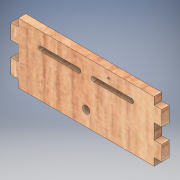
# Autodesk Inventor part: EndPulleyMount
Saved by Autodesk Inventor 2019 (Build 230136000, 136)
## iProperties
Created: 2019-01-17
Part Number: EndPulleyMount
Material: Wood (Birch)
Document SubType Name: Modeling
Designer: nxgam
Density: 0.55 g/cm^3
Appearance: Birch - Natural Polished
Author: nxgam
Autodesk Inventor part; units mm, degrees
ref_plane "YZ Plane" through (0, 0, 0) normal (1, 0, 0) x (0, 1, 0)
ref_plane "XZ Plane" through (0, 0, 0) normal (0, 1, 0) x (-1, 0, 0)
ref_plane "XY Plane" through (0, 0, 0) normal (0, 0, 1) x (1, 0, 0)
sketch "Sketch1" plane through (0, 0, 0) normal (0, 0, 1) x (1, 0, 0)
  line L0 (45.72, 0) -> (45.72, 40.64)
  line L1 (45.72, 40.64) -> (-45.72, 40.64)
  line L2 (-45.72, 40.64) -> (-45.72, 9.301)
  line L3 (-45.72, 5.08) -> (-50.8, 5.08)
  line L4 (-50.8, 5.08) -> (-50.8, 15.24)
  line L5 (-50.8, 15.24) -> (-45.72, 15.24)
  line L6 (-45.72, 15.24) -> (-45.72, 5.08)
  line L7 (-45.72, 25.4) -> (-50.8, 25.4)
  line L8 (-50.8, 25.4) -> (-50.8, 35.56)
  line L9 (-50.8, 35.56) -> (-45.72, 35.56)
  line L10 (-45.72, 35.56) -> (-45.72, 25.4)
  line L11 (-45.72, 45.72) -> (-50.8, 45.72)
  line L12 (-50.8, 45.72) -> (-50.8, 55.88)
  line L13 (-50.8, 55.88) -> (-45.72, 55.88)
  line L14 (-45.72, 55.88) -> (-45.72, 45.72)
  line L15 (0, 40.64) -> (0, 0) construction
  line L16 (45.72, 40.64) -> (45.72, 0)
  line L17 (45.72, 5.08) -> (50.8, 5.08)
  line L18 (50.8, 5.08) -> (50.8, 15.24)
  line L19 (50.8, 15.24) -> (45.72, 15.24)
  line L20 (45.72, 15.24) -> (45.72, 5.08)
  line L21 (45.72, 25.4) -> (50.8, 25.4)
  line L22 (50.8, 25.4) -> (50.8, 35.56)
  line L23 (50.8, 35.56) -> (45.72, 35.56)
  line L24 (45.72, 35.56) -> (45.72, 25.4)
  line L25 (45.72, 45.72) -> (50.8, 45.72)
  line L26 (50.8, 45.72) -> (50.8, 55.88)
  line L27 (50.8, 55.88) -> (45.72, 55.88)
  line L28 (45.72, 55.88) -> (45.72, 45.72)
  line L29 (-45.72, 5.08) -> (-45.72, 0)
  line L30 (-45.72, 0) -> (45.72, 0)
  line L31 (45.72, 40.64) -> (-45.72, 40.64)
  line L32 (-45.72, 40.64) -> (-45.72, 0)
  line L33 (-45.72, 0) -> (45.72, 0)
  line L34 (45.72, 0) -> (45.72, 40.64)
  dimension "d0" = 91.44
  dimension "d2" = 10.16
  dimension "d3" = 5.08
  dimension "d7" = 20.32
  dimension "d14" = 5.08
  dimension "d15" = 40.64
  constraints: 70 end point, 12 symmetric about line, 5 parallel, 4 perpendicular, 3 vertical, 2 horizontal, 2 midpoint, 2 point on line, 1 coincident, 16 other
  measures "d0" distance of L1.end L0.end
  measures "d2" distance of L3.end L4.end
  measures "d3" distance of L4.end L5.end
  measures "d7" distance of L3.start L7.start
  measures "d14" distance of L3.start L29.end
  measures "d15" distance between parallel lines of L30 L1
extrude "Extrusion2" add sketch "Sketch1" along normal blind 5.08 contours L30 L29 L6 L2 L1 L0 | L0 L19 L18 L17 | L3 L4 L5 L2 L6 | L0 L23 L22 L21 | L7 L8 L9 L2
sketch "Sketch4" plane through (0, 0, 5.08) normal (0, 0, 1) x (1, 0, 0)
  line L0 (45.72, 40.64) -> (-45.72, 40.64) construction
  line L1 (-30.48, 30.48) -> (-5.08, 30.48)
  line L2 (-30.48, 28.98) -> (-5.08, 28.98)
  line L3 (-5.08, 31.98) -> (-30.48, 31.98)
  arc A0 (-30.48, 31.98) -> (-30.48, 28.98) centre (-30.48, 30.48) ccw
  arc A1 (-5.08, 28.98) -> (-5.08, 31.98) centre (-5.08, 30.48) ccw
  line L4 (30.48, 30.48) -> (5.08, 30.48)
  line L5 (30.48, 28.98) -> (5.08, 28.98)
  line L6 (5.08, 31.98) -> (30.48, 31.98)
  arc A2 (30.48, 28.98) -> (30.48, 31.98) centre (30.48, 30.48) ccw
  arc A3 (5.08, 31.98) -> (5.08, 28.98) centre (5.08, 30.48) ccw
  line L7 (-50.8, 25.4) -> (-45.72, 25.4) projected
  line L8 (-45.72, 25.4) -> (-45.72, 15.24) projected
  line L9 (-45.72, 15.24) -> (-50.8, 15.24) projected
  line L10 (-50.8, 15.24) -> (-50.8, 5.08) projected
  line L11 (-50.8, 5.08) -> (-45.72, 5.08) projected
  line L12 (-45.72, 5.08) -> (-45.72, 0) projected
  line L13 (-45.72, 0) -> (45.72, 0) projected
  line L14 (45.72, 0) -> (45.72, 5.08) projected
  line L15 (45.72, 5.08) -> (50.8, 5.08) projected
  line L16 (50.8, 5.08) -> (50.8, 15.24) projected
  line L17 (50.8, 15.24) -> (45.72, 15.24) projected
  line L18 (45.72, 15.24) -> (45.72, 25.4) projected
  line L19 (45.72, 25.4) -> (50.8, 25.4) projected
  line L20 (50.8, 25.4) -> (50.8, 35.56) projected
  line L21 (50.8, 35.56) -> (45.72, 35.56) projected
  line L22 (45.72, 35.56) -> (45.72, 40.64) projected
  line L23 (45.72, 40.64) -> (-45.72, 40.64) projected
  line L24 (-45.72, 40.64) -> (-45.72, 35.56) projected
  line L25 (-45.72, 35.56) -> (-50.8, 35.56) projected
  line L26 (-50.8, 35.56) -> (-50.8, 25.4) projected
  line L27 (0, 40.64) -> (0, 0) construction
  circle A4 centre (0, 10.16) radius 2.5
  point P0 (-17.78, 30.48)
  point P1 (17.78, 30.48)
  point P2 (17.78, 30.48)
  dimension "d25" = 3
  dimension "d26" = 25.4
  dimension "d32" = 17.78
  dimension "d33" = 17.78
  dimension "d34" = 25.4
  dimension "d35" = 10.16
  dimension "d36" = 1.5
  dimension "d37" = 1.5
  dimension "d38" = 5
  dimension "d39" = 10.16
  constraints: 18 end point, 8 point on circle, 8 tangent, 5 centre point, 3 midpoint, 1 coincident, 1 collinear, 1 horizontal, 1 parallel, 1 perpendicular, 1 point on line
  measures "d25" diameter of A1
  measures "d26" distance of L1.start L1.end
  measures "d32" distance from line of point (-17.78, 30.48) L27
  measures "d33" distance from line of L27 point (17.78, 30.48)
  measures "d34" distance of L4.start L4.end
  measures "d35" distance between parallel lines of L0 L1
  measures "d36" radius of A2
  measures "d37" radius of A3
  measures "d38" diameter of A4
  measures "d39" distance from line of L13 A4.centre
extrude "Extrusion5" cut sketch "Sketch4" against normal blind 25.4 contours A0 L3 A1 L2 | L5 A3 L6 A2 | A4
equation "\"d7\" = 2 * d2"
equation "\"d33\" = d32"
equation "\"d34\" = d26"
equation "\"d36\" = 0.5 * d25"
equation "\"d37\" = d36"
equation "\"d39\" = d35"
body "Solid2"
